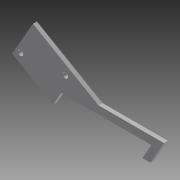
# Autodesk Inventor part: hook
Saved by Autodesk Inventor 2013 (Build 170138000, 138)
## iProperties
Created: 2013-01-24
Part Number: hook
Material: Steel
Document SubType Name: Modeling
Designer: Arpan
Density: 1 g/cm^3
Author: Arpan
Autodesk Inventor part; units mm, degrees
ref_plane "YZ Plane" through (0, 0, 0) normal (1, 0, 0) x (0, 1, 0)
ref_plane "XZ Plane" through (0, 0, 0) normal (0, 1, 0) x (-1, 0, 0)
ref_plane "XY Plane" through (0, 0, 0) normal (0, 0, 1) x (1, 0, 0)
sketch "Sketch1" plane through (0, 0, 0) normal (0, 0, 1) x (1, 0, 0)
  line L0 (0, 0) -> (130.048, 0)
  line L1 (87.9024, 12.7) -> (59.6729, 12.7)
  line L2 (87.9024, 12.7) -> (130.048, 12.7)
  line L3 (130.048, 12.7) -> (130.048, 0)
  line L4 (130.048, -25.4) -> (142.748, -25.4)
  line L5 (130.048, -25.4) -> (144.7127, 0)
  line L6 (142.748, -25.4) -> (164.745, 12.7)
  line L7 (144.7127, 0) -> (130.048, 0)
  line L8 (130.048, 12.7) -> (164.745, 12.7)
  line L9 (0, 0) -> (7.3323, 12.7)
  line L10 (3.6662, 6.35) -> (20.4175, 35.3641)
  line L11 (3.6662, 6.35) -> (-13.0851, -22.6641)
  line L12 (-13.0851, -22.6641) -> (-78.9003, 15.3343)
  line L13 (-78.9003, 15.3343) -> (-45.3977, 73.3625)
  line L14 (-45.3977, 73.3625) -> (20.4175, 35.3641)
  line L15 (20.4175, 35.3641) -> (59.6729, 12.7)
  line L16 (20.4175, 35.3641) -> (13.4893, 39.3641)
  circle A0 centre (6.7393, 27.6728) radius 4.15
  line L17 (-78.9003, 15.3343) -> (-71.9721, 11.3343)
  circle A1 centre (-65.2221, 23.0256) radius 4.1529
  dimension "d39" = 130.048
  dimension "d41" = 25.4
  dimension "d42" = 12.7
  dimension "d43" = 60
  dimension "d44" = 60
  dimension "d45" = 12.7
  dimension "d51" = 136.3234
  dimension "d54" = 136.3234
  dimension "d55" = 12.7
  dimension "d56" = 66.5476
  dimension "d57" = 33.5026
  dimension "d58" = 33.5026
  dimension "d59" = 75.9968
  dimension "d60" = 40.8349
  dimension "d61" = 8
  dimension "d63" = 8.3
  dimension "d64" = 8
  dimension "d66" = 8.3058
  constraints: 36 end point, 4 parallel, 3 collinear, 3 perpendicular, 3 point on line, 2 centre point, 2 horizontal, 1 midpoint
  measures "d39" distance of L0.start L0.end
  measures "d41" distance of L0.end L4.start
  measures "d42" distance of L4.start L4.end
  measures "d43" angle of L5 L4
  measures "d44" angle of L4 L6
  measures "d45" distance between parallel lines of L1 L0
  measures "d51" distance between parallel lines of L6 L9
  measures "d54" distance from line of point (0, 0) L6
  measures "d55" distance from line of point (0, 0) L8
  measures "d56" distance from line of L1.start L6
  measures "d57" distance of L10.start L10.end
  measures "d58" distance of L10.start L11.end
  measures "d59" distance of L11.end L12.end
  measures "d60" distance from line of point (0, 0) L14
  measures "d61" distance of L10.end L16.end
  measures "d63" diameter of A0
  measures "d64" distance of L12.end L17.end
  measures "d66" diameter of A1
extrude "Extrusion1" add sketch "Sketch1" along normal blind 6.35
body "Solid1"
